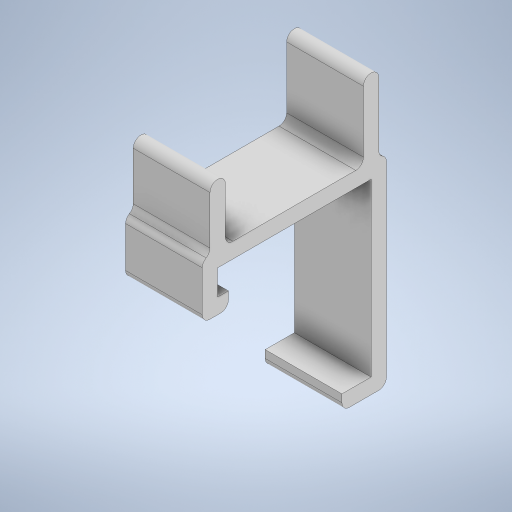
# Autodesk Inventor part: monitor-clip
Saved by Autodesk Inventor 2023 (Build 270158030, 158C)
## iProperties
Created: 2024-02-28
Part Number: monitor-clip
Material: Generic
Document SubType Name: Modeling
Designer: Imogen Heard
Density: 1 g/cm^3
Appearance: Default
Author: Imogen Heard
Autodesk Inventor part; units mm, degrees
ref_plane "YZ Plane" through (0, 0, 0) normal (1, 0, 0) x (0, 1, 0)
ref_plane "XZ Plane" through (0, 0, 0) normal (0, 1, 0) x (-1, 0, 0)
ref_plane "XY Plane" through (0, 0, 0) normal (0, 0, 1) x (1, 0, 0)
sketch "Sketch1" plane through (0, 0, 0) normal (1, 0, 0) x (0, 1, 0)
  line L0 (10.279, 12) -> (9.5154, 12)
  line L1 (9.5154, 12) -> (9.5154, 10.3)
  line L2 (9.5154, 10.3) -> (10.5154, 10.3)
  line L3 (10.5154, 10.3) -> (10.5154, 11)
  line L4 (10.5154, 11) -> (12.1654, 11)
  line L5 (13.1654, 12) -> (10.279, 12)
  line L6 (13.1654, 12) -> (13.1654, 1)
  line L7 (12.1654, 1) -> (12.1654, 11)
  line L8 (12.1654, 1) -> (1, 1)
  line L9 (0, 1.2006) -> (0, 0)
  line L10 (0, 0) -> (13.1654, 0)
  line L11 (13.1654, 0) -> (13.1654, 1)
  line L12 (0, 1.2006) -> (0, 2.9)
  line L13 (0, 2.9) -> (1, 2.9)
  line L14 (1, 2.9) -> (1, 1)
  dimension "d0" = 0.7
  dimension "d1" = 1.65
  dimension "d2" = 10
  dimension "d3" = 11.1654
  dimension "d4" = 1
  dimension "d5" = 1
  dimension "d6" = 1
  dimension "d7" = 1
  dimension "d8" = 1
  dimension "d9" = 1.9
  constraints: 30 end point, 7 parallel, 3 horizontal, 2 perpendicular, 2 point on line, 1 coincident
  measures "d0" distance between parallel lines of L2 L4
  measures "d1" distance between parallel lines of L7 L3
  measures "d2" distance between parallel lines of L8 L4
  measures "d3" distance between parallel lines of L14 L7
  measures "d4" distance between parallel lines of L1 L3
  measures "d5" distance between parallel lines of L4 L5
  measures "d6" distance between parallel lines of L7 L6
  measures "d7" distance between parallel lines of L10 L8
  measures "d8" distance between parallel lines of L12 L14
  measures "d9" distance between parallel lines of L8 L13
extrude "Extrusion1" add sketch "Sketch1" along normal blind 5
fillet "Fillet1" radius 0.5 6 edges at (2.5, 9.5154, 10.3) (2.5, 9.5154, 12) (2.5, 13.1654, 12) (2.5, 13.1654, 0) (2.5, 0, 0) (2.5, 0, 2.9)
sketch "Sketch2" plane through (5, 0, 0) normal (1, 0, 0) x (0, 0, -1)
  line L0 (-0.5, 13.1654) -> (-11.5, 13.1654) projected
  line L1 (-11.5, 13.1654) -> (-10.5, 13.1654)
  line L2 (-10.5, 13.1654) -> (-10.5, 17.1654)
  line L3 (-10.5, 17.1654) -> (-11.5, 17.1654)
  line L4 (-11.5, 17.1654) -> (-11.5, 13.1654)
  line L5 (-0.5, 18.1654) -> (-1.5, 18.1654)
  line L6 (-1.5, 18.1654) -> (-1.5, 13.1654)
  line L7 (-1.5, 13.1654) -> (-0.5, 13.1654)
  line L8 (-0.5, 13.1654) -> (-0.5, 18.1654)
  point P0 (0, 0)
  dimension "d13" = 10
  dimension "d14" = 1
  dimension "d15" = 1
  dimension "d16" = 5
  dimension "d17" = 4
  constraints: 16 end point, 4 parallel, 2 coincident, 2 horizontal, 2 perpendicular, 2 point on line
  measures "d13" distance between parallel lines of L8 L2
  measures "d14" distance between parallel lines of L2 L4
  measures "d15" distance between parallel lines of L6 L8
  measures "d16" distance between parallel lines of L0 L5
  measures "d17" distance between parallel lines of L0 L3
extrude "Extrusion2" add sketch "Sketch2" against normal blind 5
fillet "Fillet2" radius 0.5 8 edges at (2.5, 13.1654, 10.5) (2.5, 13.1654, 11.5) (2.5, 17.1654, 11.5) (2.5, 17.1654, 10.5) (2.5, 13.1654, 1.5) (2.5, 18.1654, 1.5) (2.5, 18.1654, 0.5) (2.5, 13.1654, 0.5)
body "Solid1"
